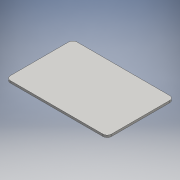
# Autodesk Inventor part: sampleHolderXYstageBase
Saved by Autodesk Inventor 2016 (Build 200138000, 138)
## iProperties
Created: 2016-11-09
Part Number: sampleHolderXYstageBase
Material: Generic
Document SubType Name: Modeling
Designer: sims01
Density: 1 g/cm^3
Appearance: Default
Author: sims01
Autodesk Inventor part; units mm, degrees
ref_plane "YZ Plane" through (0, 0, 0) normal (1, 0, 0) x (0, 1, 0)
ref_plane "XZ Plane" through (0, 0, 0) normal (0, 1, 0) x (-1, 0, 0)
ref_plane "XY Plane" through (0, 0, 0) normal (0, 0, 1) x (1, 0, 0)
sketch "Sketch1" plane through (0, 0, 0) normal (0, 0, 1) x (1, 0, 0)
  line L0 (-75.75, 54.75) -> (75.75, 54.75)
  line L1 (79.75, 50.75) -> (79.75, -50.75)
  line L2 (75.75, -54.75) -> (-75.75, -54.75)
  line L3 (-79.75, -50.75) -> (-79.75, 50.75)
  arc A0 (-75.75, 54.75) -> (-79.75, 50.75) centre (-75.75, 50.75) ccw
  arc A1 (-79.75, -50.75) -> (-75.75, -54.75) centre (-75.75, -50.75) ccw
  arc A2 (75.75, -54.75) -> (79.75, -50.75) centre (75.75, -50.75) ccw
  arc A3 (79.75, 50.75) -> (75.75, 54.75) centre (75.75, 50.75) ccw
  point P0 (0, 0)
  point P1 (-79.75, 54.75)
  point P2 (79.75, -54.75)
  point P3 (79.75, 54.75)
  dimension "d0" = 159.5
  dimension "d1" = 79.75
  dimension "d2" = 109.5
  dimension "d3" = 54.75
  dimension "d4" = 4
  constraints: 8 end point, 8 point on circle, 8 tangent, 6 point on line, 4 centre point, 3 equal radius, 2 parallel, 1 horizontal, 1 perpendicular
  measures "d0" distance of point (-79.75, 54.75) point (79.75, 54.75)
  measures "d1" distance from line of point (0, 0) L1
  measures "d2" distance of point (79.75, 54.75) point (79.75, -54.75)
  measures "d3" distance from line of point (0, 0) L0
  measures "d4" radius of A0
extrude "Extrusion1" add sketch "Sketch1" along normal blind 3
sketch "Sketch2" plane through (0, 0, 3) normal (0, 0, 1) x (1, 0, 0)
  line L0 (-109.1, 78.6) -> (109.1, 78.6)
  line L1 (119.1, 68.6) -> (119.1, -68.6)
  line L2 (109.1, -78.6) -> (-109.1, -78.6)
  line L3 (-119.1, -68.6) -> (-119.1, 68.6)
  arc A0 (-109.1, 78.6) -> (-119.1, 68.6) centre (-109.1, 68.6) ccw
  arc A1 (-119.1, -68.6) -> (-109.1, -78.6) centre (-109.1, -68.6) ccw
  arc A2 (109.1, -78.6) -> (119.1, -68.6) centre (109.1, -68.6) ccw
  arc A3 (119.1, 68.6) -> (109.1, 78.6) centre (109.1, 68.6) ccw
  point P0 (0, 0)
  point P1 (-119.1, 78.6)
  point P2 (119.1, 78.6)
  point P3 (-119.1, -78.6)
  dimension "d7" = 238.2
  dimension "d8" = 157.2
  dimension "d9" = 119.1
  dimension "d10" = 78.6
  dimension "d11" = 10
  constraints: 8 end point, 8 point on circle, 8 tangent, 6 point on line, 4 centre point, 3 equal radius, 2 parallel, 1 horizontal, 1 perpendicular
  measures "d7" distance of point (-119.1, 78.6) point (119.1, 78.6)
  measures "d8" distance of point (-119.1, -78.6) point (-119.1, 78.6)
  measures "d9" distance from line of point (0, 0) L1
  measures "d10" distance from line of point (0, 0) L0
  measures "d11" radius of A0
extrude "Extrusion2" add sketch "Sketch2" along normal blind 5
equation "\"d1\" = 0.5 * d0"
equation "\"d3\" = 0.5 * d2"
equation "\"d9\" = 0.5 * d7"
equation "\"d10\" = 0.5 * d8"
body "Solid1"
